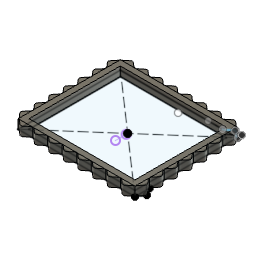
BottomCasePanelWavy v2 (Autodesk Fusion 360 design; units mm, degrees)
Autodesk Fusion 360 part; units mm, degrees
note: some values were not read from the file. Chosen so that the rebuilt part matches the saved one: which face or edge a step refers to. Set by a fixed rule: which sketch regions a step uses.
sketch "Sketch1" plane through (0, 0, 0) normal (0, 1, 0) x (1, 0, 0)
  line L0 (-96, 84) -> (96.1411, 84)
  spline S0 degree 5 poles (96.1411, 84) (95.6964, 84) (94.7833, 84.1504) (93.3428, 84.827) (91.3133, 86.4829) (88.7656, 89.0171) (86.3472, 91.087) (84.1411, 91.9006) (81.9351, 91.087) (79.5167, 89.0171) (76.969, 86.4829) (74.9395, 84.827) (73.499, 84.1504) (72.5859, 84) (72.1411, 84) knots 0 0 0 0 0 0 0.1 0.2 0.3 0.4 0.5 0.6 0.7 0.8 0.9 1 1 1 1 1 1
  line L1 (98.6411, 91.5) -> (69.6411, 91.5)
  line L2 (96.1411, 84) -> (48.1411, 84) construction
  line L3 (96.1411, 84) -> (96.1411, 91.5) construction
  line L4 (110.6411, 84) -> (81.6411, 84)
  line L5 (86.6411, 84) -> (57.6411, 84)
  line L6 (0, -20) -> (0, -2.5) construction
  line L7 (96, -84) -> (-96, -84)
  line L8 (-96, -84) -> (-96, 84)
  line L9 (-96, 84) -> (96, 84)
  line L10 (96, 84) -> (96, -84)
  line L11 (96, -84) -> (-96, 84) construction
  line L12 (-96, -84) -> (96, 84) construction
  line L13 (-87, 75) -> (87, 75)
  line L14 (87, 75) -> (87, -75)
  line L15 (87, -75) -> (-87, -75)
  line L16 (-87, -75) -> (-87, 75)
  spline S1 degree 5 poles (96.1411, 84) (95.6721, 84) (94.7267, 84.1704) (93.2865, 84.9372) (91.3325, 86.814) (88.8865, 89.686) (86.4808, 92.0319) (84.1411, 92.954) (81.8015, 92.0319) (79.3958, 89.686) (76.9498, 86.814) (74.9958, 84.9372) (73.5556, 84.1704) (72.6102, 84) (72.1411, 84) knots 0 0 0 0 0 0 0.1 0.2 0.3 0.4 0.5 0.6 0.7 0.8 0.9 1 1 1 1 1 1
  line L17 (110.6411, 84) -> (81.6411, 84)
  line L18 (98.6411, 92.5) -> (69.6411, 92.5)
  line L19 (86.6411, 84) -> (57.6411, 84)
  spline S2 degree 5 poles (96.1411, 84) (95.6721, 84) (94.7267, 84.1704) (93.2865, 84.9372) (91.3325, 86.814) (88.8865, 89.686) (86.4808, 92.0319) (84.1411, 92.954) (81.8015, 92.0319) (79.3958, 89.686) (76.9498, 86.814) (74.9958, 84.9372) (73.5556, 84.1704) (72.6102, 84) (72.1411, 84) knots 0 0 0 0 0 0 0.1 0.2 0.3 0.4 0.5 0.6 0.7 0.8 0.9 1 1 1 1 1 1
  line L20 (110.6411, 84) -> (81.6411, 84)
  line L21 (98.6411, 92.5) -> (69.6411, 92.5)
  line L22 (86.6411, 84) -> (57.6411, 84)
  spline S3 degree 5 poles (96, -84) (96, -83.5553) (96.1504, -82.6421) (96.827, -81.2016) (98.4829, -79.1722) (101.0171, -76.6244) (103.087, -74.206) (103.9006, -72) (103.087, -69.794) (101.0171, -67.3756) (98.4829, -64.8278) (96.827, -62.7984) (96.1504, -61.3579) (96, -60.4447) (96, -60) knots 0 0 0 0 0 0 0.1 0.2 0.3 0.4 0.5 0.6 0.7 0.8 0.9 1 1 1 1 1 1
  line L23 (96, -98.5) -> (96, -69.5)
  line L24 (103.5, -86.5) -> (103.5, -57.5)
  line L25 (96, -74.5) -> (96, -45.5)
  point P0 (84.1411, 91.5)
  point P1 (96.1411, 91.5)
  point P2 (84.1411, 91.5)
  point P3 (12, 70.903)
  point P4 (84.1411, 92.5)
  point P5 (84.1411, 92.5)
  point P6 (103.5, -72)
  dimension "d37" = 12
  dimension "d38" = 7.5
  dimension "d40" = 12
  dimension "d43" = 29
  dimension "d46" = 29
  dimension "d47" = 29
  dimension "d55" = 168
  dimension "d56" = 192
  dimension "d65" = 9
  dimension "d68" = 29
  dimension "d69" = 29
  dimension "d70" = 29
  dimension "d71" = 29
  dimension "d72" = 29
  dimension "d73" = 29
  dimension "d74" = 29
  dimension "d75" = 29
  dimension "d76" = 29
  dimension "d77" = 7.5
  dimension "d78" = 12
  dimension "d79" = 12
  constraint horizontal L0
  constraint coincident L0 S0.end
  constraint midpoint P2 L1
  constraint coincident P2 P0
  constraint coincident P1 L3.end
  constraint vertical L3
  constraint midpoint L0.end L4
  constraint midpoint S0.end L5
  constraint coincident L2 L5.end
  constraint parallel L2 L5
  constraint coincident L0 L4.end
  constraint horizontal L7
  constraint perpendicular L7 L8
  constraint parallel L7 L9
  constraint parallel L8 L10
  constraint coincident L11 origin
  constraint coincident L12 origin
  constraint coincident L1 P1
  constraint midpoint P5 L18
  constraint midpoint L0.end L17
  constraint midpoint S0.end L19
  constraint midpoint P5 L21
  constraint midpoint L0.end L20
  constraint midpoint S0.end L22
  constraint midpoint P6 L24
  constraint midpoint L7.start L23
  constraint midpoint S3.end L25
  constraint vertical L25
  constraint vertical L23
  constraint vertical L24
  constraint coincident L10 S3.end
  measures "d37" distance of P1 P2
  measures "d38" distance of L0.end L3.end
  measures "d40" distance of S0.end P2
  measures "d43" distance of L1.start L1.end
  measures "d46" distance of L5.start L5.end
  measures "d47" distance of L4.start L4.end
  measures "d55" distance of L7.start L9.end
  measures "d56" distance of L7.start L7.end
  measures "d68" distance of L18.end L18.start
  measures "d69" distance of L5.end L5.start
  measures "d70" distance of L4.end L4.start
  measures "d71" distance of L18.end L18.start
  measures "d72" distance of L5.end L5.start
  measures "d73" distance of L4.end L4.start
  measures "d74" distance of L24.end L24.start
  measures "d75" distance of L25.end L25.start
  measures "d76" distance of L23.end L23.start
  measures "d77" distance of S3.end L24
  measures "d78" vertical distance of L7.start P6
  measures "d79" distance of P6 S3.end
extrude "Extrude1" add sketch "Sketch1" along normal blind 15 contours L0 L4 L5 L7 L8 L9 L10 L17 L19 L20 L22 L23 L25 makes body 1
extrude "Extrude2" add sketch "Sketch1" along normal up to surface (15 mm away) separate body contours L0 S0 L4 L5 L9 L17 L19 L20 L22 | L10 S3 L23 L25 makes body 2 at (93.5823, 12.8571, -84.8557) makes body 3 at (96.8557, 12.8571, 81.4412)
pattern_linear "R-Pattern1" count 8 spacing 24 along (-1, 0, 0) of bodies 2 makes body 4 at (69.5823, 12.8571, -84.8557) makes body 5 at (45.5823, 12.8571, -84.8557) makes body 6 at (21.5823, 12.8571, -84.8557) makes body 7 at (-2.4177, 12.8571, -84.8557) makes body 8 at (-26.4177, 12.8571, -84.8557) makes body 9 at (-50.4177, 12.8571, -84.8557) makes body 10 at (-74.4177, 12.8571, -84.8557)
mirror "Mirror2" about plane through (0, 0, 0) normal (0, 0, 1) of bodies 2 4 5 6 7 8 9 10 makes body 11 at (93.5823, 12.8571, 84.8557) makes body 12 at (69.5823, 12.8571, 84.8557) makes body 13 at (45.5823, 12.8571, 84.8557) makes body 14 at (21.5823, 12.8571, 84.8557) makes body 15 at (-2.4177, 12.8571, 84.8557) makes body 16 at (-26.4177, 12.8571, 84.8557) makes body 17 at (-50.4177, 12.8571, 84.8557) makes body 18 at (-74.4177, 12.8571, 84.8557)
pattern_linear "R-Pattern2" count 7 spacing 24 along (0, 0, -1) of bodies 3 makes body 19 at (96.8557, 12.8571, 57.4412) makes body 20 at (96.8557, 12.8571, 33.4412) makes body 21 at (96.8557, 12.8571, 9.4412) makes body 22 at (96.8557, 12.8571, -14.5588) makes body 23 at (96.8557, 12.8571, -38.5588) makes body 24 at (96.8557, 12.8571, -62.5588)
mirror "Mirror3" about plane through (0, 0, 0) normal (1, 0, 0) of bodies 3 19 20 21 22 23 24 makes body 25 at (-96.8557, 12.8571, 81.4412) makes body 26 at (-96.8557, 12.8571, 57.4412) makes body 27 at (-96.8557, 12.8571, 33.4412) makes body 28 at (-96.8557, 12.8571, 9.4412) makes body 29 at (-96.8557, 12.8571, -14.5588) makes body 30 at (-96.8557, 12.8571, -38.5588) makes body 31 at (-96.8557, 12.8571, -62.5588)
sketch "Sketch3" plane through (0, 0, 0) normal (0, 1, 0) x (1, 0, 0)
  line L0 (60, -37.5) -> (-60, -37.5)
  line L1 (-60, -37.5) -> (-60, 37.5)
  line L2 (-60, 37.5) -> (60, 37.5)
  line L3 (60, 37.5) -> (60, -37.5)
  line L4 (60, -37.5) -> (-60, 37.5) construction
  line L5 (-60, -37.5) -> (60, 37.5) construction
  dimension "d66" = 75
  dimension "d67" = 120
  constraint horizontal L0
  constraint perpendicular L0 L1
  constraint parallel L0 L2
  constraint parallel L1 L3
  constraint coincident L4 origin
  constraint coincident L5 origin
  measures "d66" distance of L0.end L1.end
  measures "d67" distance of L1.end L2.end
equation "SideWidth = 9 mm"
equation "d5 = PanelHeights"
equation "CaseHeight = 75 mm"
equation "CaseLength = 192 mm"
equation "CaseWidth = 168 mm"
equation "PanelHeights = 15 mm"
equation "d37 = CaseLength / 16"
equation "WaveWidth = 20 mm"
equation "d40 = CaseLength / 16"
equation "d43 = WaveControlLength"
equation "d46 = WaveControlLength"
equation "d47 = WaveControlLength"
equation "WaveControlLength = 29 mm"
equation "d55 = CaseWidth"
equation "d56 = CaseLength"
equation "d61 = -CaseLength + CaseLength / 8"
equation "d65 = SideWidth"
equation "d68 = WaveControlLength"
equation "d69 = WaveControlLength"
equation "d70 = WaveControlLength"
equation "d71 = WaveControlLength"
equation "d72 = WaveControlLength"
equation "d73 = WaveControlLength"
equation "d74 = WaveControlLength"
equation "d75 = WaveControlLength"
equation "d76 = WaveControlLength"
equation "d78 = CaseWidth / 14"
equation "d79 = CaseWidth / 14"
equation "d84 = -CaseWidth + CaseWidth / 7"
